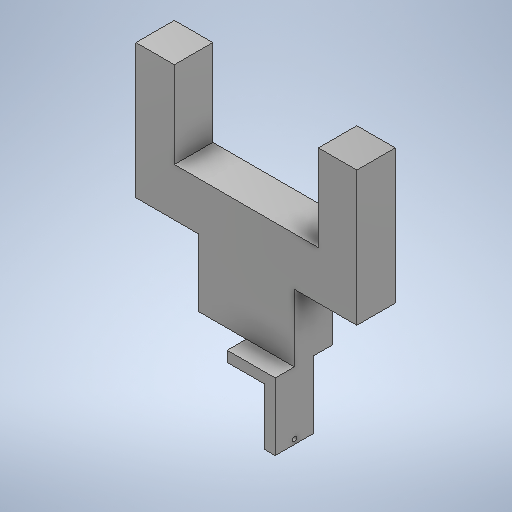
# Autodesk Inventor part: Robot_arm_gripper
Saved by Autodesk Inventor 2025 (Build 290162010, 162A)
## iProperties
Created: 2024-07-13
Part Number: Robot_arm_gripper
Material: Generic
Document SubType Name: Modeling
Designer: saees
Density: 1 g/cm^3
Appearance: Anodized - Light Gray
Author: saees
Autodesk Inventor part; units mm, degrees
ref_plane "YZ Plane" through (0, 0, 0) normal (1, 0, 0) x (0, 1, 0)
ref_plane "XZ Plane" through (0, 0, 0) normal (0, 1, 0) x (-1, 0, 0)
sketch "Sketch1" plane through (0, 0, 0) normal (0, 0, 1) x (1, 0, 0)
  line L0 (-50, 0) -> (-50, 70)
  line L1 (-50, 70) -> (-115, 70)
  line L2 (-115, 70) -> (-115, 210)
  line L3 (-115, 210) -> (-75, 210)
  line L4 (-75, 210) -> (-75, 120)
  line L5 (-75, 120) -> (75, 120)
  line L6 (75, 120) -> (75, 210)
  line L7 (75, 210) -> (115, 210)
  line L8 (115, 210) -> (115, 70)
  line L9 (115, 70) -> (50, 70)
  line L10 (50, 70) -> (50, 0)
  line L11 (50, 0) -> (-50, 0)
  point P0 (0, 0)
  point P1 (0, 120)
  point P2 (0, 0)
  dimension "d0" = 100
  dimension "d1" = 150
  dimension "d2" = 40
  dimension "d3" = 140
  dimension "d4" = 90
  dimension "d5" = 70
  constraints: 24 end point, 9 perpendicular, 4 point on line, 2 midpoint, 1 coincident, 1 collinear, 1 vertical, 1 vertical alignment
  measures "d0" distance of L10.end L0.start
  measures "d1" distance of L4.end L5.end
  measures "d2" distance of L2.end L3.end
  measures "d3" distance of L1.end L2.end
  measures "d4" distance of L3.end L4.end
  measures "d5" distance of L9.end L10.end
extrude "Extrusion1" add sketch "Sketch1" along normal blind 40
sketch "Sketch2" plane through (-50, 0, 0) normal (0, -1, 0) x (1, 0, 0)
  line L0 (0, 0) -> (0, 40) projected
  line L1 (100, 0) -> (100, 40) projected
  line L2 (0, 40) -> (100, 40) projected
  circle A0 centre (50, 20) radius 2.5
  point P0 (50, 0)
  dimension "d8" = 5
  constraints: 1 centre point
  measures "d8" diameter of A0
extrude "Extrusion2" cut sketch "Sketch2" against normal blind 40
ref_plane "Work Plane1" through (0, 0, 20) normal (0, 0, 1) x (1, 0, 0)
sketch "Sketch3" plane through (0, 0, 20) normal (0, 0, 1) x (1, 0, 0)
  line L0 (-50, 0) -> (50, 0) projected
  line L1 (0, 0) -> (50, 0)
  line L2 (50, 0) -> (50, -70)
  line L3 (50, -70) -> (39.0685, -70)
  line L4 (39.0685, -70) -> (39.0685, -10.9315)
  line L5 (39.0685, -10.9315) -> (0, -10.9315)
  line L6 (0, -10.9315) -> (0, 0)
  dimension "d12" = 70
  dimension "d13" = 39.0685
  constraints: 12 end point, 6 perpendicular, 1 collinear
  measures "d12" distance of L0.end L2.end
  measures "d13" distance of L4.end L5.end
extrude "Extrusion3" add sketch "Sketch3" along normal blind 40
sketch "Sketch4" plane through (50, 0, 0) normal (1, 0, 0) x (0, 0, -1)
  circle A0 centre (-40, -65) radius 2.5
  line L0 (-20, -70) -> (-60, -70) projected
  point P0 (0, 0)
  point P1 (-40, -70)
  point P2 (-40, -70)
  dimension "d16" = 5
  dimension "d17" = 5
  constraints: 2 midpoint, 1 centre point, 1 vertical alignment
  measures "d16" diameter of A0
  measures "d17" distance of point (-40, -70) A0.centre
extrude "Extrusion4" cut sketch "Sketch4" against normal blind 40
body "Solid1"
